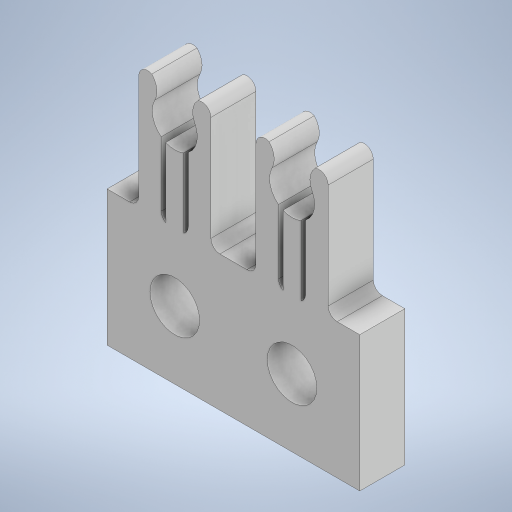
# Autodesk Inventor part: Test fuse holder
Saved by Autodesk Inventor 2024 (Build 280153000, 153)
## iProperties
Created: 2024-04-04
Part Number: Test fuse holder
Material: Generic
Document SubType Name: Modeling
Designer: jens1
Density: 1 g/cm^3
Appearance: Default
Author: jens1
Autodesk Inventor part; units mm, degrees
ref_plane "YZ Plane" through (0, 0, 0) normal (1, 0, 0) x (0, 1, 0)
ref_plane "XZ Plane" through (0, 0, 0) normal (0, 1, 0) x (-1, 0, 0)
ref_plane "XY Plane" through (0, 0, 0) normal (0, 0, 1) x (1, 0, 0)
sketch "Sketch1" plane through (0, 0, 0) normal (0, 0, 1) x (1, 0, 0)
  point P0 (0, 0)
sketch "Sketch2" plane through (0, 0, 0) normal (0, 0, 1) x (1, 0, 0)
  line L0 (0, 0) -> (28, 0)
  line L1 (28, 0) -> (28, 15)
  line L2 (28, 15) -> (0, 15)
  line L3 (0, 15) -> (0, 0)
  line L4 (3.5, 15) -> (3.5, 27.6125)
  line L5 (6, 15) -> (6, 23)
  line L6 (9, 15) -> (9, 23)
  line L7 (11.5, 15) -> (11.5, 27.6125)
  circle A0 centre (7.5, 25) radius 2.25
  circle A1 centre (7.5, 25) radius 2.5
  line L8 (6.5, 15) -> (6.5, 22.7087)
  line L9 (8.5, 15) -> (8.5, 22.7087)
  line L10 (4.9567, 28.5021) -> (7.4, 27.2478)
  line L11 (10.0433, 28.5021) -> (7.6, 27.2478)
  arc A2 (4.9567, 28.5021) -> (3.5, 27.6125) centre (4.5, 27.6125) ccw
  arc A3 (11.5, 27.6125) -> (10.0433, 28.5021) centre (10.5, 27.6125) ccw
  line L12 (0, 0) -> (14, 0)
  line L13 (14, 0) -> (14, 15)
  line L14 (14, 15) -> (0, 15)
  line L15 (0, 15) -> (0, 0)
  line L16 (24.5, 15) -> (24.5, 27.6125)
  line L17 (22, 15) -> (22, 23)
  line L18 (19, 15) -> (19, 23)
  line L19 (16.5, 15) -> (16.5, 27.6125)
  circle A4 centre (20.5, 25) radius 2.25
  circle A5 centre (20.5, 25) radius 2.5
  line L20 (21.5, 15) -> (21.5, 22.7087)
  line L21 (19.5, 15) -> (19.5, 22.7087)
  line L22 (23.0433, 28.5021) -> (20.6, 27.2478)
  line L23 (17.9567, 28.5021) -> (20.4, 27.2478)
  arc A6 (24.5, 27.6125) -> (23.0433, 28.5021) centre (23.5, 27.6125) ccw
  arc A7 (17.9567, 28.5021) -> (16.5, 27.6125) centre (17.5, 27.6125) ccw
  point P0 (3.5, 29.25)
  point P1 (11.5, 29.25)
  point P2 (20.9949, 27.4505)
  point P3 (20.0051, 27.4505)
  point P4 (7.9949, 27.4505)
  point P5 (7.0051, 27.4505)
  dimension "d0" = 28
  dimension "d1" = 15
  dimension "d2" = 4.5
  dimension "d3" = 5
  dimension "d4" = 3.5
  dimension "d5" = 2.5
  dimension "d6" = 2
  dimension "d7" = 1
  dimension "d8" = 2.5
  dimension "d9" = 0.5
  dimension "d10" = 0.5
  dimension "d11" = 0
  dimension "d12" = 0.2
  dimension "d13" = 14.25
  dimension "d14" = 14.25
  dimension "d15" = 10
  dimension "d16" = 1
  dimension "d17" = 14
  dimension "d18" = 15
  constraints: 48 end point, 20 point on circle, 20 symmetric about line, 10 point on line, 8 centre point, 8 parallel, 4 tangent, 2 coincident, 2 horizontal, 2 perpendicular, 2 vertical, 1 equal radius, 4 other
  measures "d0" distance of L2.end L1.end
  measures "d1" distance of L1.end L0.end
  measures "d2" diameter of A0
  measures "d3" diameter of A1
  measures "d4" distance between parallel lines of L4 L3
  measures "d5" distance between parallel lines of L5 L4
  measures "d6" distance between parallel lines of L9 L8
  measures "d7" distance from line of L8 A0.centre
  measures "d8" distance between parallel lines of L7 L6
  measures "d9" distance between parallel lines of L9 L6
  measures "d10" distance between parallel lines of L8 L5
  measures "d11" vertical distance of L10.end L11.end
  measures "d12" distance of L10.end L11.end
  measures "d13" distance of L4.start point (3.5, 29.25)
  measures "d14" distance of L7.start point (11.5, 29.25)
  measures "d15" distance from line of L2 A1.centre
  measures "d16" radius of A2
  measures "d17" distance of L14.end L13.end
  measures "d18" distance of L13.end L12.end
extrude "Extrusion1" add sketch "Sketch2" along normal blind 5 contours L3 L2 L13 L0 | L13 L2 L1 L0 | L4 A2 L10 A1 L5 L2 | L19 A7 L23 A5 L18 L2 | L2 L6 A1 L11 A3 L7 | L2 L17 A5 L22 A6 L16 | L8 A1 L9 L2 | L21 A5 L20 L2
fillet "Fillet1" radius 2 4 edges at (7.0051, 27.4505, 2.5) (20.0051, 27.4505, 2.5) (7.9949, 27.4505, 2.5) (20.9949, 27.4505, 2.5)
fillet "Fillet2" radius 1 8 edges at (3.5, 15, 2.5) (6, 15, 2.5) (9, 15, 2.5) (11.5, 15, 2.5) (16.5, 15, 2.5) (19, 15, 2.5) (22, 15, 2.5) (24.5, 15, 2.5)
sketch "Sketch3" plane through (0, 0, 5) normal (0, 0, 1) x (1, 0, 0)
  line L0 (2.5, 15) -> (0, 15) projected
  line L1 (0, 0) -> (28, 0) projected
  line L2 (0, 15) -> (28, 15)
  line L3 (28, 15) -> (28, 0)
  line L4 (28, 0) -> (0, 0)
  line L5 (0, 0) -> (0, 15)
  arc A0 (6.5, 22.7087) -> (8.5, 22.7087) centre (7.5, 25) ccw projected
  arc A1 (19.5, 22.7087) -> (21.5, 22.7087) centre (20.5, 25) ccw projected
  point P0 (7.5, 7.5)
  point P1 (20.5, 7.5)
  dimension "d23" = 0
  dimension "d24" = 0
  dimension "d25" = 0
  dimension "d26" = 15
  dimension "d27" = 7.5
  constraints: 8 end point, 2 parallel, 1 horizontal, 1 perpendicular
  measures "d23" vertical distance of point (20.5, 7.5) point (7.5, 7.5)
  measures "d24" horizontal distance of A0.centre point (7.5, 7.5)
  measures "d25" horizontal distance of A1.centre point (20.5, 7.5)
  measures "d26" distance of L2.end L1.end
  measures "d27" distance from line of L2 point (20.5, 7.5)
hole "Hole1" at (7.5, 7.5, 5) at (20.5, 7.5, 5) direction (0, 0, -1) diameter 5.5 end through all
equation "\"d14\" = d13"
equation "\"d18\" = d1"
equation "\"d27\" = 0.5 * d26"
body "Solid1"
